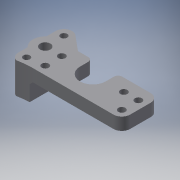
# Autodesk Inventor part: BLTouch_Connector_joined
Saved by Autodesk Inventor 2016 (Build 200138000, 138)
## iProperties
Created: 2015-12-28
Part Number: BLTouch_Connector_joined
Material: Generic
Document SubType Name: Modeling
Designer: inornate
Density: 1 g/cm^3
Appearance: Default
Author: inornate
Autodesk Inventor part; units mm, degrees
ref_plane "YZ Plane" through (0, 0, 0) normal (1, 0, 0) x (0, 1, 0)
ref_plane "XZ Plane" through (0, 0, 0) normal (0, 1, 0) x (-1, 0, 0)
ref_plane "XY Plane" through (0, 0, 0) normal (0, 0, 1) x (1, 0, 0)
sketch "Sketch1" plane through (0, 0, 0) normal (0, 0, 1) x (1, 0, 0)
  circle A0 centre (-18.3043, -1.4966) radius 1.7
  circle A1 centre (18.6957, -1.4966) radius 1.7
  circle A2 centre (18.6957, 6.5034) radius 1.7 projected
  circle A3 centre (-18.3043, 6.5034) radius 1.7 projected
  circle A4 centre (11.6957, 6.5034) radius 1.7 projected
  arc A5 (22.6957, 8.5034) -> (18.6957, 12.5034) centre (18.6957, 8.5034) ccw
  line L0 (4.8957, 12.5034) -> (18.6957, 12.5034)
  arc A6 (4.8957, 12.5034) -> (2.8957, 10.5034) centre (4.8957, 10.5034) ccw
  line L1 (2.8957, 6.5034) -> (2.8957, 10.5034)
  arc A7 (-9.5043, 6.5034) -> (2.8957, 6.5034) centre (-3.3043, 6.5034) ccw projected
  line L2 (-9.5043, 10.5034) -> (-9.5043, 6.5034)
  arc A8 (-9.5043, 10.5034) -> (-11.5043, 12.5034) centre (-11.5043, 10.5034) ccw
  line L3 (-16.508, 12.5034) -> (-11.5043, 12.5034)
  line L4 (18.6957, -5.4966) -> (-18.3043, -5.4966)
  circle A9 centre (-18.3043, 6.5034) radius 1.7 projected
  circle A10 centre (-26.3043, -2.4966) radius 1.6 projected
  circle A11 centre (-26.3043, 15.5034) radius 1.6 projected
  line L5 (-23.3147, 18.1609) -> (-16.508, 12.5034)
  arc A12 (-23.3147, 18.1609) -> (-30.3043, 15.5034) centre (-26.3043, 15.5034) ccw projected
  line L6 (-30.3043, 10.9756) -> (-30.3043, 15.5034) projected
  arc A13 (-30.3043, 10.9756) -> (-30.3043, 2.0313) centre (-26.3043, 6.5034) ccw projected
  line L7 (-30.3043, -2.4966) -> (-30.3043, 2.0313) projected
  arc A14 (-30.3043, -2.4966) -> (-27.7088, -6.2419) centre (-26.3043, -2.4966) ccw projected
  circle A15 centre (-26.3043, 6.5034) radius 2.5 projected
  arc A16 (-18.3043, -5.4966) -> (-27.7088, -6.2419) centre (-19.7185, -47.358) ccw
  line L8 (22.6957, 8.5034) -> (22.6957, -1.4966)
  arc A17 (18.6957, -5.4966) -> (22.6957, -1.4966) centre (18.6957, -1.4966) ccw
  point P0 (0, 0)
  point P1 (-18.3043, 6.5034)
  dimension "d14" = 12
  dimension "d17" = 8
  dimension "d18" = 4
  dimension "d24" = 6
  dimension "d25" = 2
  dimension "d26" = 2
  dimension "d27" = 2
  dimension "d28" = 2
  constraints: 14 end point, 10 point on circle, 7 centre point, 2 horizontal, 2 horizontal alignment, 2 parallel, 2 vertical alignment, 1 collinear, 1 tangent
  measures "d14" distance from line of L4 A7.centre
  measures "d17" distance of point (-18.304, 6.503) A0.centre
  measures "d18" radius of A17
  measures "d24" distance from line of L0 A7.centre
  measures "d25" distance from line of L3 A8.centre
  measures "d26" distance from line of L2 A8.centre
  measures "d27" radius of A6
  measures "d28" distance from line of A6.centre L1
extrude "Extrusion1" add sketch "Sketch1" against normal blind 6
sketch "Sketch2" plane through (0, 0, -6) normal (0, 0, -1) x (-1, 0, 0)
  circle A0 centre (26.3043, -2.4966) radius 1.6 projected
  circle A1 centre (26.3043, 15.5034) radius 1.6 projected
  circle A2 centre (26.3043, 6.5034) radius 2.5 projected
  arc A3 (30.3043, 15.5034) -> (23.3147, 18.1609) centre (26.3043, 15.5034) ccw projected
  circle A4 centre (18.3043, 6.5034) radius 1.7 projected
  circle A5 centre (18.3043, -5.4966) radius 1.7 projected
  circle A6 centre (26.3043, -2.4966) radius 1.6 projected
  circle A7 centre (26.3043, 15.5034) radius 1.6 projected
  line L0 (14.3043, 6.5034) -> (14.3043, -5.4966) projected
  arc A8 (14.3043, -5.4966) -> (19.7088, -9.2419) centre (18.3043, -5.4966) ccw projected
  line L1 (19.7088, -9.2419) -> (27.7088, -6.2419) projected
  arc A9 (27.7088, -6.2419) -> (30.3043, -2.4966) centre (26.3043, -2.4966) ccw projected
  line L2 (30.3043, -2.4966) -> (30.3043, 2.0313) projected
  arc A10 (30.3043, 2.0313) -> (30.3043, 10.9756) centre (26.3043, 6.5034) ccw projected
  line L3 (30.3043, 10.9756) -> (30.3043, 15.5034) projected
  arc A11 (30.3043, 15.5034) -> (23.3147, 18.1609) centre (26.3043, 15.5034) ccw projected
  line L4 (23.3147, 18.1609) -> (15.3147, 9.1609) projected
  arc A12 (15.3147, 9.1609) -> (14.3043, 6.5034) centre (18.3043, 6.5034) ccw projected
  line L5 (18.3043, 12.5242) -> (23.3147, 18.1609) construction
  arc A13 (27.7088, -6.2419) -> (18.3043, -5.4966) centre (19.7185, -47.358) ccw projected
  line L6 (23.3147, 18.1609) -> (16.508, 12.5034) projected
  line L7 (-4.8957, 12.5034) -> (-18.6957, 12.5034) projected
  line L8 (21.8043, 16.9055) -> (21.8043, -5.5246)
  line L9 (25.163, -7.1966) -> (21.8043, -5.5246)
  circle A14 centre (18.3043, 6.5034) radius 1.7 projected
  point P0 (0, 0)
  dimension "d22" = 3.5
  constraints: 6 end point, 2 point on line, 2 tangent, 1 coincident, 1 perpendicular, 1 point on circle, 3 other
  measures "d22" distance from line of L8 A14.centre
extrude "Extrusion2" add sketch "Sketch2" along normal blind 9 contours L3 A10 L2 A9 A13 L8 L4 A3 | L4 L8 L6
chamfer "Chamfer1" distance 1.5 angle 45 1 edges at (-21.8043, 5.6904, -6)
sketch "Sketch4" plane through (0, 0, -6) normal (0, 0, -1) x (-1, 0, 0)
  circle A0 centre (-11.6957, 6.5034) radius 1.7 projected
  circle A1 centre (18.3043, 6.5034) radius 1.7 projected
  line L0 (-8.4337, 6.5034) -> (-10.0647, 3.6784)
  line L1 (-10.0647, 3.6784) -> (-13.3267, 3.6784)
  line L2 (-13.3267, 3.6784) -> (-14.9577, 6.5034)
  line L3 (-14.9577, 6.5034) -> (-13.3267, 9.3284)
  line L4 (-13.3267, 9.3284) -> (-10.0647, 9.3284)
  line L5 (-10.0647, 9.3284) -> (-8.4337, 6.5034)
  line L6 (15.0423, 6.5034) -> (16.6733, 9.3284)
  line L7 (16.6733, 9.3284) -> (19.9353, 9.3284)
  line L8 (19.9353, 9.3284) -> (21.5663, 6.5034)
  line L9 (21.5663, 6.5034) -> (19.9353, 3.6784)
  line L10 (19.9353, 3.6784) -> (16.6733, 3.6784)
  line L11 (16.6733, 3.6784) -> (15.0423, 6.5034)
  dimension "d21" = 5.65
  constraints: 24 end point, 2 coincident, 1 collinear, 26 other
  measures "d21" distance between parallel lines of L1 L4
extrude "Extrusion3" cut sketch "Sketch4" against normal blind 3 and the other way blind 5
body "Solid1"
